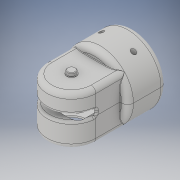
# Autodesk Inventor part: Thigh-40x
Saved by Autodesk Inventor 2018 (Build 220112000, 112)
## iProperties
Created: 2017-08-15
Part Number: Thigh-40x
Material: Generisch
Document SubType Name: Modeling
Designer: JochenAlt
Density: 1 g/cm^3
Appearance: Vorgabe
Mass: 57.7164 g
Surface Area: 269.653 cm^2
Volume: 57.7164 cm^3
Author: JochenAlt
Autodesk Inventor part; units mm, degrees
ref_plane "YZ Plane" through (0, 0, 0) normal (1, 0, 0) x (0, 1, 0)
ref_plane "XZ Plane" through (0, 0, 0) normal (0, 1, 0) x (-1, 0, 0)
ref_plane "Arbeitsebene2" through (0, 0, 0) normal (0, 0, 1) x (1, 0, 0)
sketch "Skizze Herkulex 040x" plane through (0, 0, 0) normal (0, 0, 1) x (1, 0, 0)
  line L0 (0, -49.2432) -> (0, 42.9739) construction
  line L1 (-28.937, 0) -> (28.937, 0) construction
  line L2 (14.8, 28.3) -> (-14.8, 28.3)
  line L3 (-17.8, 25.3) -> (-17.8, -22.3)
  line L4 (-11.8, -28.3) -> (11.8, -28.3)
  line L5 (17.8, -22.3) -> (17.8, 25.3)
  line L6 (17.8, 28.3) -> (-17.8, -28.3) construction
  line L7 (-17.8, 28.3) -> (17.8, -28.3) construction
  arc A0 (-17.8, -22.3) -> (-11.8, -28.3) centre (-11.8, -22.3) ccw
  arc A1 (11.8, -28.3) -> (17.8, -22.3) centre (11.8, -22.3) ccw
  arc A2 (17.8, 25.3) -> (14.8, 28.3) centre (14.8, 25.3) ccw
  arc A3 (-14.8, 28.3) -> (-17.8, 25.3) centre (-14.8, 25.3) ccw
  line L8 (8.5, 21.2) -> (-8.5, 21.2)
  line L9 (-11.5, 18.2) -> (-11.5, -25.3)
  line L10 (-8.5, -28.3) -> (8.5, -28.3)
  line L11 (11.5, -25.3) -> (11.5, 18.2)
  line L12 (11.5, 21.2) -> (-11.5, -28.3) construction
  line L13 (-11.5, 21.2) -> (11.5, -28.3) construction
  arc A4 (-11.5, -25.3) -> (-8.5, -28.3) centre (-8.5, -25.3) ccw
  arc A5 (-8.5, 21.2) -> (-11.5, 18.2) centre (-8.5, 18.2) ccw
  arc A6 (11.5, 18.2) -> (8.5, 21.2) centre (8.5, 18.2) ccw
  arc A7 (8.5, -28.3) -> (11.5, -25.3) centre (8.5, -25.3) ccw
  circle A8 centre (0, -15.4) radius 12.75
  circle A9 centre (-13.5, 23.5) radius 1
  circle A10 centre (13.5, 23.5) radius 1
  line L14 (-13.5, -22.4) -> (13.5, -22.4) construction
  line L15 (13.5, -22.4) -> (13.5, 23.5) construction
  line L16 (13.5, 23.5) -> (-13.5, 23.5) construction
  line L17 (-13.5, 23.5) -> (-13.5, -22.4) construction
  line L18 (5.5, -8.75) -> (-5.5, -8.75) construction
  line L19 (5.5, -18.5) -> (-5.5, -18.5)
  line L20 (-5.5, 1) -> (5.5, 1)
  arc A11 (5.5, -18.5) -> (5.5, 1) centre (5.5, -8.75) ccw
  arc A12 (-5.5, 1) -> (-5.5, -18.5) centre (-5.5, -8.75) ccw
  circle A13 centre (0, -15.4) radius 4
  line L21 (-20.6693, 29.8) -> (20.6693, 29.8)
  line L22 (-20.6693, 29.8) -> (-20.6693, -15.4)
  line L23 (20.6693, -15.4) -> (20.6693, 29.8)
  arc A14 (-20.6693, -15.4) -> (20.6693, -15.4) centre (0, -15.4) ccw
  circle A15 centre (-13.5, 23.5) radius 2
  circle A16 centre (13.5, 23.5) radius 2
  arc A17 (14, -23.6) -> (14, -21.2) centre (14, -22.4) ccw construction
  arc A18 (14, -21.2) -> (14, -23.6) centre (14, -22.4) ccw construction
  arc A19 (-14, -21.2) -> (-14, -23.6) centre (-14, -22.4) ccw construction
  arc A20 (-14, -23.6) -> (-14, -21.2) centre (-14, -22.4) ccw construction
  circle A21 centre (14, -22.4) radius 1
  circle A22 centre (-14, -22.4) radius 1
  circle A23 centre (0, 15) radius 10
  point P0 (0, 0)
  point P1 (0, -3.55)
  point P2 (0, -8.75)
  dimension "d115" = 35.6
  dimension "d116" = 56.6
  dimension "d117" = 6
  dimension "d118" = 49.5
  dimension "d119" = 23
  dimension "d120" = 3
  dimension "d121" = 25.5
  dimension "d122" = 15.4
  dimension "d124" = 2
  dimension "d125" = 2
  dimension "d128" = 45.9
  dimension "d129" = 7
  dimension "d130" = 19.5
  dimension "d131" = 30.5
  dimension "d132" = 8
  dimension "d163" = 1.5
  dimension "d167" = 1
  dimension "d169" = 4
  dimension "d170" = 4
  dimension "d171" = 27
  dimension "d219" = 2
  dimension "d220" = 2
  dimension "d221" = 3
  dimension "d222" = 3
  dimension "d223" = 3
  dimension "d224" = 1
  dimension "d225" = 20
  dimension "d226" = 15
  constraints: 46 end point, 30 point on circle, 24 centre point, 22 point on line, 22 tangent, 8 parallel, 6 midpoint, 5 coincident, 4 perpendicular, 3 concentric, 3 horizontal, 2 equal radius, 1 collinear, 1 vertical, 13 other
  measures "d115" distance of L7.end L6.end
  measures "d116" distance of L6.end L7.start
  measures "d117" radius of A0
  measures "d118" distance between parallel lines of L8 L10
  measures "d119" distance between parallel lines of L11 L9
  measures "d120" radius of A4
  measures "d121" diameter of A8
  measures "d122" distance of A8.centre point (0, 0)
  measures "d124" diameter of A9
  measures "d125" diameter of A10
  measures "d128" distance between parallel lines of L16 L14
  measures "d129" distance from line of A8.centre L14
  measures "d130" distance between parallel lines of L20 L19
  measures "d132" diameter of A13
  measures "d163" distance between parallel lines of L21 L2
  measures "d169" diameter of A15
  measures "d170" diameter of A16
  measures "d171" distance between parallel lines of L15 L17
  measures "d219" diameter of A21
  measures "d220" diameter of A22
  measures "d221" radius of A2
  measures "d222" radius of A3
  measures "d223" radius of A6
  measures "d224" distance between parallel lines of L1 L20
  measures "d225" diameter of A23
  measures "d226" distance from line of L1 A23.centre
extrude "Extrusion1" add sketch "Skizze Herkulex 040x" against normal blind 31.9 contours A2 L5 A1 L4 A7 L11 A8 A11 A6 L8 A23 A5 L9 A12 A4 A0 L3 A3 L2 | L4 A4 L9 A8 L11 A7 | A8 L9 A12 L19 A13 A11 L11 | L11 A11 A8 | A8 A12 L9 | A11 L19 A13 A12 L9 A8 L11 | L11 A8 A11 | A12 A8 L9 | A12 L9 A8 | A8 L9 A12 L20 A11 L11 | L11 A11 A8 | L9 A5 L8 A23 A6 L11 A11 L20 A12 | A13 L19 | L19 A13 | A23 L8 | L8 A23 | A9 | A10 | A15 | A16 | A21 | A22
fillet "Rundung11" radius 1 16 edges at (-16.0426, -26.5426, 0) (-17.8, 1.5, 0) (-16.9213, 27.4213, 0) (0, 28.3, 0) (16.9213, 27.4213, 0) (17.8, 1.5, 0) (16.0426, -26.5426, 0) (0, -28.3, 0) (0, -28.3, -31.9) (-16.0426, -26.5426, -31.9) (-17.8, 1.5, -31.9) (-16.9213, 27.4213, -31.9) (0, 28.3, -31.9) (16.9213, 27.4213, -31.9) (17.8, 1.5, -31.9) (16.0426, -26.5426, -31.9)
extrude "Extrusion2" add sketch "Skizze Herkulex 040x" along normal blind 3 contours L4 A4 L9 A8 L11 A7 | A8 L9 A12 L19 A13 A11 L11 | A11 L19 A13 A12 L9 A8 L11 | L11 A8 A11 | A12 A8 L9 | A12 L9 A8 | A8 L9 A12 L20 A11 L11 | L11 A11 A8 | L9 A5 L8 A23 A6 L11 A11 L20 A12 | A13 L19 | L19 A13 | A23 L8 | L8 A23 picked at (11.7255, -12.6495) picked at (-11.7255, -12.6495) picked at (-12.0402, -4.5424) picked at (12.0402, -4.5424)
extrude "Extrusion3" add sketch "Skizze Herkulex 040x" against normal blind 35 contours L4 A4 L9 A8 L11 A7 | A8 L9 A12 L19 A13 A11 L11 | A11 L19 A13 A12 L9 A8 L11 | L11 A8 A11 | A12 A8 L9 | A12 L9 A8 | A8 L9 A12 L20 A11 L11 | L11 A11 A8 | L9 A5 L8 A23 A6 L11 A11 L20 A12 | A13 L19 | L19 A13 | A23 L8 | L8 A23 picked at (11.7255, -12.6495) picked at (-11.7255, -12.6495) picked at (-12.0402, -4.5424) picked at (12.0402, -4.5424)
extrude "Extrusion4" add sketch "Skizze Herkulex 040x" against normal blind 50 contours A8 L9 A12 L19 A13 A11 L11 | L11 A11 A8 | A8 A12 L9 | A11 L19 A13 A12 L9 A8 L11 | L11 A8 A11 | A12 A8 L9 | A13 L19 | L19 A13 picked at (11.7298, -18.8268) picked at (-11.734, -18.813) picked at (11.7255, -12.6495) picked at (-11.7255, -12.6495)
extrude "Extrusion5" add sketch "Skizze Herkulex 040x" against normal blind 36.4 and the other way blind 4.6 separate body contours A2 L5 A1 L4 A7 L11 A8 A11 A6 L8 A23 A5 L9 A12 A4 A0 L3 A3 L2 | L4 A4 L9 A8 L11 A7 | A8 L9 A12 L19 A13 A11 L11 | L11 A11 A8 | A8 A12 L9 | A11 L19 A13 A12 L9 A8 L11 | L11 A8 A11 | A12 A8 L9 | A12 L9 A8 | A8 L9 A12 L20 A11 L11 | L11 A11 A8 | L9 A5 L8 A23 A6 L11 A11 L20 A12 | A13 L19 | L19 A13 | A23 L8 | L8 A23 | A9 | A10 | L21 L23 A14 L22 | A15 | A16 | A21 | A22
sketch "Skizze4" plane through (-23.6693, 29.8, -36.4) normal (0, 1, 0) x (1, 0, 0)
  line L0 (3, 0) -> (44.3386, -41) construction
  line L1 (44.3386, -41) -> (44.3386, 0) construction
  line L2 (44.3386, 0) -> (1.4042, -41) construction
  circle A0 centre (22.8714, -20.5) radius 28
  dimension "d168" = 56
  constraints: 4 end point, 1 centre point, 1 midpoint
  measures "d168" diameter of A0
sketch "Skizze Lagerflansch" plane through (0, -16.4396, 4.6) normal (0, 0, 1) x (1, 0, 0)
  circle A0 centre (0, 1.0239) radius 4
  circle A1 centre (0, 1.0239) radius 3.4
  point P0 (0, 16.4396)
  dimension "d73" = 8
  dimension "d76" = 6.8
  constraints: 2 centre point, 1 coincident
  measures "d73" diameter of A0
  measures "d76" diameter of A1
extrude "Extrusion Lagerflansch" add sketch "Skizze Lagerflansch" along normal blind 0.5 contours A0 | A1 bodies 2
extrude "Extrusion Lagerachse" add sketch "Skizze Lagerflansch" along normal blind 3 contours A1 bodies 2
chamfer "Fase8" distance 0.5 angle 45 1 edges at (-3.4, -15.4157, 7.6)
fillet "Rundung3" radius 4.1 6 edges at (0, -36.0693, -36.4) (20.6693, 7.2, -36.4) (-20.6693, 7.2, -36.4) (0, -36.0693, 4.6) (20.6693, 7.2, 4.6) (-20.6693, 7.2, 4.6)
extrude "Extrusion6" add sketch "Skizze4" along normal blind 8.3 and the other way blind 25 bodies 2
combine bodies "Kombinieren1" operation type subtract main body 2 bodies to subtract 1
ref_plane "Trennfläche" through (-0.7979, 29.8, -15.9) normal (0, 0, 1) x (1, 0, 0)
sketch "Skizze16" plane through (-0.7979, 0.1, -15.9) normal (0, 0, 1) x (1, 0, 0)
  line L0 (33.5581, -15.4) -> (-28.6036, -15.4)
  line L1 (-28.6036, -15.4) -> (-28.6036, -48.1191)
  line L2 (-28.6036, -48.1191) -> (33.5581, -48.1191)
  line L3 (33.5581, -48.1191) -> (33.5581, -15.4)
  line L4 (-28.6036, -63.6829) -> (-28.6036, 45.2638) construction
  line L5 (-41.036, -0.1) -> (45.9904, -0.1) construction
  point P0 (0.7979, -0.1)
  point P1 (-28.6036, 45.2638)
  point P2 (-20.6693, -15.4)
  constraints: 8 end point, 2 parallel, 1 horizontal, 1 perpendicular, 1 point on line, 1 vertical, 3 other
extrude "Extrusion20" cut sketch "Skizze16" along normal blind 5 bodies 2
fillet "Rundung9" radius 2 4 edges at (19.2347, -15.3, -10.9) (19.2347, -15.3, -15.9) (-19.2347, -15.3, -10.9) (-19.2347, -15.3, -15.9)
fillet "Rundung10" radius 2 6 edges at (0, -36.0693, -15.9) (20.6592, -16.0478, -15.4595) (20.6693, -15.3252, -12.5838) (20.6693, -15.3252, -14.2162) (20.6592, -16.0477, -11.3406) (0, -36.0693, -10.9)
fillet "Rundung4" radius 5 1 edges at (-28.7979, 4.8, -15.9)
fillet "Rundung5" radius 0.5 19 edges at (-20.6693, 4.9798, -29.9362) (-19.4789, 6.6122, -35.1886) (-16.5696, 5.7022, -36.4) (-13.9479, 4.9871, -36.4) (-0.7979, 4.8, -36.4) (13.2655, 5.1589, -36.4) (19.4267, 9.3952, -35.2402) (20.6693, 5.1552, -28.4188) (20.6693, 4.8, -15.9) (20.6693, 5.1551, -3.3814) (20.6693, 6.8197, 0.4998) (19.4383, 9.4022, 3.429) (13.2657, 5.159, 4.6) (-0.7979, 4.8, 4.6) (-13.9479, 4.9871, 4.6) (-20.6693, 5.634, 0.4999) (-19.4772, 6.6123, 3.3904) (-20.6693, 4.9798, -1.8639) (-20.6693, 4.8, -15.9)
sketch "Skizze5" plane through (-0.7979, 38.1, -15.9) normal (0, 1, 0) x (1, 0, 0)
  circle A0 centre (0, 0) radius 21
  point P0 (0.7979, -15.9)
  dimension "d54" = 42
  constraints: 1 centre point
  measures "d54" diameter of A0
extrude "Extrusion7" cut sketch "Skizze5" against normal blind 1.2 bodies 2
sketch "Skizze6" plane through (-0.7979, 36.9, -15.9) normal (0, 1, 0) x (1, 0, 0)
  circle A0 centre (0, 0) radius 22.4
  point P0 (0.7979, -15.9)
  dimension "d57" = 44.8
  constraints: 1 centre point
  measures "d57" diameter of A0
extrude "Extrusion8" cut sketch "Skizze6" against normal blind 5.2 bodies 2
sketch "Skizze7" plane through (-0.7979, 31.7, -15.9) normal (0, 1, 0) x (1, 0, 0)
  circle A0 centre (0, 0) radius 20.5
  point P0 (0.7979, -15.9)
  dimension "d60" = 41
  constraints: 1 centre point
  measures "d60" diameter of A0
extrude "Extrusion9" cut sketch "Skizze7" against normal blind 1.5 bodies 2
sketch "Skizze8" plane through (-0.7979, 30.2, -15.9) normal (0, 1, 0) x (1, 0, 0)
  line L0 (-39.2, -15.9) -> (39.2, -15.9) construction
  line L1 (0.7979, 39.2) -> (0.7979, -39.2) construction
  line L2 (10.8103, 9.2843) -> (10.8103, -9.2843)
  arc A0 (10.8103, 9.2843) -> (-10.8103, 9.2843) centre (0, 0) ccw
  arc A1 (-10.8103, -9.2843) -> (10.8103, -9.2843) centre (0, 0) ccw
  line L3 (-10.8103, 9.2843) -> (-10.8103, -9.2843)
  circle A2 centre (0, 0) radius 20.5 projected
  line L4 (10.8103, -9.2843) -> (-10.8103, 9.2843) construction
  line L5 (-10.8103, -9.2843) -> (10.8103, 9.2843) construction
  point P0 (0.7979, -15.9)
  point P1 (0, 0)
  dimension "d237" = 14.25
  dimension "d238" = 14.25
  constraints: 8 end point, 5 point on circle, 2 centre point, 2 midpoint, 1 concentric, 1 vertical
  measures "d237" radius of A0
  measures "d238" radius of A1
extrude "Extrusion10" add sketch "Skizze8" along normal blind 1.5 contours L2 A1 L3 A0 bodies 2
sketch "Skizze9" plane through (-0.7979, 31.7, -15.9) normal (0, 1, 0) x (1, 0, 0)
  circle A0 centre (0, 0) radius 8
  point P0 (0.7979, -15.9)
  dimension "d67" = 16
  constraints: 1 centre point
  measures "d67" diameter of A0
extrude "Extrusion11" cut sketch "Skizze9" against normal up to next bodies 2
sketch "Skizze22" plane through (-0.7979, 29.8, -15.9) normal (0, 0, 1) x (1, 0, 0)
  line L0 (3.8176, 0.4) -> (15.5979, 0.4)
  line L1 (20.0979, -4.1) -> (20.0979, -48.0928)
  arc A0 (20.0979, -4.1) -> (15.5979, 0.4) centre (15.5979, -4.1) ccw
  line L2 (20.0979, -48.0928) -> (3.8176, -48.0928)
  line L3 (3.8176, 0.4) -> (3.8176, -48.0928)
  arc A1 (18.5979, -4.5) -> (15.5979, -1.5) centre (15.5979, -4.5) ccw construction
  arc A2 (-17.0021, -52.1) -> (-11.0021, -58.1) centre (-11.0021, -52.1) ccw construction
  line L4 (-17.0021, -4.5) -> (-17.0021, -52.1) construction
  line L5 (-18.5021, -55.5259) -> (-18.5021, -4.5)
  line L6 (-17.0021, -4.5) -> (-18.5021, -4.5)
  line L7 (-17.0021, -54.4699) -> (-18.5021, -54.4699)
  line L8 (-17.0021, -4.5) -> (-17.0021, -54.4699)
  line L9 (-18.5021, -10.1) -> (20.0979, -10.1)
  line L10 (20.0979, -10.1) -> (20.0979, -21.1)
  line L11 (20.0979, -21.1) -> (-18.5021, -21.1)
  line L12 (-18.5021, -21.1) -> (-18.5021, -10.1)
  line L13 (9.2979, -58.1) -> (-7.7021, -58.1) projected
  dimension "d211" = 4.5
  dimension "d239" = 3
  dimension "d240" = 1.5
  dimension "d241" = 37
  dimension "d243" = 11
  constraints: 24 end point, 4 horizontal, 3 parallel, 3 point on circle, 2 perpendicular, 2 point on line, 2 tangent, 1 centre point, 1 collinear, 1 vertical, 5 other
  measures "d211" radius of A0
  measures "d239" radius of A1
  measures "d240" distance between parallel lines of L5 L4
  measures "d241" distance between parallel lines of L13 L11
  measures "d243" distance between parallel lines of L11 L9
extrude "Extrusion24" cut sketch "Skizze22" along normal blind 5 contours L0 A0 L1 L9 L3 | L9 L1 L11 L3 | L11 L1 L2 L3 | L9 L5 L6 L8 | L8 L11 L5 L9 | L8 L7 L5 L11 bodies 2
extrude "Extrusion26" cut sketch "Skizze22" against normal blind 7 contours L9 L1 L11 L3 | L3 L11 L8 L9 | L8 L11 L5 L9 bodies 2
fillet "Rundung6" radius 5 1 edges at (-28.7979, 38.1, -15.9)
sketch "Skizze14" plane through (-16.1, 28.3, 0) normal (0, -1, 0) x (1, 0, 0)
  line L0 (6.3021, -6.9) -> (24.3021, -6.9)
  line L1 (24.3021, -6.9) -> (24.3021, -24.9)
  line L2 (24.3021, -24.9) -> (6.3021, -24.9)
  line L3 (6.3021, -24.9) -> (6.3021, -6.9)
  line L4 (6.3021, -6.9) -> (24.3021, -24.9) construction
  line L5 (24.3021, -6.9) -> (6.3021, -24.9) construction
  line L6 (32.4654, -8.2) -> (-2.5346, -8.2)
  line L7 (-2.5346, -8.2) -> (-2.5346, -18.2)
  line L8 (-2.5346, -18.2) -> (32.4654, -18.2)
  line L9 (32.4654, -18.2) -> (32.4654, -8.2)
  line L10 (32.4654, -8.2) -> (-2.5346, -18.2) construction
  line L11 (-2.5346, -8.2) -> (32.4654, -18.2) construction
  circle A0 centre (15.3021, -15.9) radius 28 construction
  point P0 (16.1, 0)
  point P1 (14.9654, -13.2)
  point P2 (16, 0)
  point P3 (16, 0)
  point P4 (16, 0)
  dimension "d98" = 18
  dimension "d99" = 18
  dimension "d102" = 10
  dimension "d103" = 8.2
  dimension "d104" = 35
  constraints: 24 end point, 4 midpoint, 4 parallel, 2 horizontal, 2 perpendicular, 1 coincident
  measures "d98" distance of L1.end L2.end
  measures "d99" distance of L0.end L1.end
  measures "d102" distance between parallel lines of L6 L8
  measures "d103" distance from line of point (16.1, 0) L6
  measures "d104" distance between parallel lines of L7 L9
extrude "Extrusion19" cut sketch "Skizze14" against normal blind 2.2 contours L0 L1 L6 L3 | L6 L1 L8 L3 | L8 L1 L2 L3 bodies 2
extrude "Extrusion16" cut sketch "Skizze Herkulex 040x" along normal through all both and the other way through all contours A9 | A10 bodies 2
extrude "Extrusion17" cut sketch "Skizze Herkulex 040x" against normal blind 7 from surface at -35 contours A9 | A10 | A15 | A16 bodies 2
extrude "Extrusion18" cut sketch "Skizze Herkulex 040x" along normal blind 20 from surface at 3 contours A9 | A10 | A15 | A16 bodies 2
chamfer "Fase18" distance 0.5 angle 45 2 edges at (-21.2979, 31.7, -15.9) (-21.7979, 36.9, -15.9)
split body "Trennen3" result two bodies by plane through (-0.7979, 29.8, -15.9) normal (0, 0, 1) bodies 2 first body at (5.5296, 22.0953, 10.8622)
sketch "Skizze21" plane through (-0.7979, 29.8, -15.9) normal (0, 0, 1) x (1, 0, 0)
  point P0 (0.7979, -29.8)
